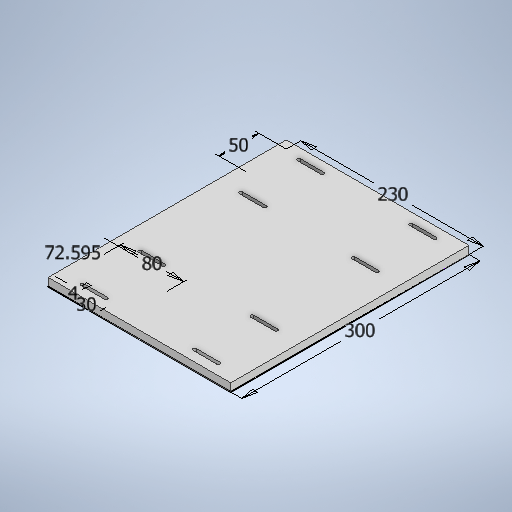
# Autodesk Inventor part: base
Saved by Autodesk Inventor 2025.3 (Build 293356030, 356C)
## iProperties
Created: 2026-06-25
Part Number: base
Material: Generic
Document SubType Name: Modeling
Designer: user
Density: 1 g/cm^3
Appearance: Default
Author: user
Autodesk Inventor part; units mm, degrees
ref_plane "YZ Plane" through (0, 0, 0) normal (1, 0, 0) x (0, 1, 0)
ref_plane "XZ Plane" through (0, 0, 0) normal (0, 1, 0) x (-1, 0, 0)
ref_plane "XY Plane" through (0, 0, 0) normal (0, 0, 1) x (1, 0, 0)
sketch "Sketch1" plane through (0, 0, 0) normal (0, 1, 0) x (-1, 0, 0)
  line L0 (0, 0) -> (-230, 0)
  line L1 (-230, 0) -> (-230, -300)
  line L2 (-230, -300) -> (0, -300)
  line L3 (0, -300) -> (0, 0)
  line L4 (-115, 0) -> (-115, -300) construction
  line L5 (-230, -150) -> (0, -150) construction
  line L6 (0, -250) -> (-230, -250) construction
  line L7 (0, -28.043) -> (0, -96.333) construction
  line L8 (0, -69) -> (0, -31) construction
  line L9 (0, -50) -> (-230, -50) construction
  line L10 (0, -31) -> (-80, -31) construction
  line L11 (-80, -31) -> (-80, -69) construction
  line L12 (-80, -69) -> (0, -69) construction
  line L13 (0, -69) -> (0, -31)
  line L14 (-40, -50) -> (-40, -10.0475) construction
  line L15 (-40, -13.7025) -> (-29.2216, -13.7025)
  line L16 (-40, -13.7025) -> (-59.2216, -13.7025)
  line L17 (-29.2216, -13.7025) -> (-59.2216, -13.7025) construction
  line L18 (-29.2216, -11.7025) -> (-59.2216, -11.7025)
  line L19 (-59.2216, -15.7025) -> (-29.2216, -15.7025)
  arc A0 (-29.2216, -15.7025) -> (-29.2216, -11.7025) centre (-29.2216, -13.7025) ccw
  arc A1 (-59.2216, -11.7025) -> (-59.2216, -15.7025) centre (-59.2216, -13.7025) ccw
  line L20 (-40, -86.2975) -> (-29.2216, -86.2975)
  line L21 (-40, -86.2975) -> (-59.2216, -86.2975)
  line L22 (-29.2216, -86.2975) -> (-59.2216, -86.2975) construction
  line L23 (-29.2216, -88.2975) -> (-59.2216, -88.2975)
  line L24 (-59.2216, -84.2975) -> (-29.2216, -84.2975)
  arc A2 (-29.2216, -88.2975) -> (-29.2216, -84.2975) centre (-29.2216, -86.2975) ccw
  arc A3 (-59.2216, -84.2975) -> (-59.2216, -88.2975) centre (-59.2216, -86.2975) ccw
  line L25 (-230, -31) -> (-150, -31) construction
  line L26 (-150, -31) -> (-150, -69) construction
  line L27 (-150, -69) -> (-230, -69) construction
  line L28 (-190, -13.7025) -> (-200.7784, -13.7025)
  line L29 (-190, -13.7025) -> (-170.7784, -13.7025)
  line L30 (-200.7784, -13.7025) -> (-170.7784, -13.7025) construction
  line L31 (-200.7784, -11.7025) -> (-170.7784, -11.7025)
  line L32 (-170.7784, -15.7025) -> (-200.7784, -15.7025)
  arc A4 (-200.7784, -11.7025) -> (-200.7784, -15.7025) centre (-200.7784, -13.7025) ccw
  arc A5 (-170.7784, -15.7025) -> (-170.7784, -11.7025) centre (-170.7784, -13.7025) ccw
  arc A6 (-170.7784, -88.2975) -> (-170.7784, -84.2975) centre (-170.7784, -86.2975) ccw
  line L33 (-190, -86.2975) -> (-170.7784, -86.2975)
  line L34 (-170.7784, -84.2975) -> (-200.7784, -84.2975)
  line L35 (-190, -86.2975) -> (-200.7784, -86.2975)
  line L36 (-200.7784, -86.2975) -> (-170.7784, -86.2975) construction
  line L37 (-200.7784, -88.2975) -> (-170.7784, -88.2975)
  arc A7 (-200.7784, -84.2975) -> (-200.7784, -88.2975) centre (-200.7784, -86.2975) ccw
  line L38 (-115, -300) -> (-115, 0) construction
  line L39 (0, -250) -> (-230, -250) construction
  line L40 (0, -269) -> (-80, -269) construction
  line L41 (-80, -269) -> (-80, -231) construction
  line L42 (-80, -231) -> (0, -231) construction
  line L43 (-40, -250) -> (-40, -289.9525) construction
  line L44 (-40, -286.2975) -> (-29.2216, -286.2975)
  line L45 (-40, -286.2975) -> (-59.2216, -286.2975)
  line L46 (-29.2216, -286.2975) -> (-59.2216, -286.2975) construction
  line L47 (-29.2216, -288.2975) -> (-59.2216, -288.2975)
  line L48 (-59.2216, -284.2975) -> (-29.2216, -284.2975)
  arc A8 (-29.2216, -288.2975) -> (-29.2216, -284.2975) centre (-29.2216, -286.2975) ccw
  arc A9 (-59.2216, -284.2975) -> (-59.2216, -288.2975) centre (-59.2216, -286.2975) ccw
  arc A10 (-59.2216, -211.7025) -> (-59.2216, -215.7025) centre (-59.2216, -213.7025) ccw
  line L49 (-40, -213.7025) -> (-59.2216, -213.7025)
  line L50 (-59.2216, -215.7025) -> (-29.2216, -215.7025)
  line L51 (-40, -213.7025) -> (-29.2216, -213.7025)
  line L52 (-29.2216, -213.7025) -> (-59.2216, -213.7025) construction
  line L53 (-29.2216, -211.7025) -> (-59.2216, -211.7025)
  arc A11 (-29.2216, -215.7025) -> (-29.2216, -211.7025) centre (-29.2216, -213.7025) ccw
  line L54 (-150, -269) -> (-150, -231) construction
  line L55 (-170.7784, -284.2975) -> (-200.7784, -284.2975)
  line L56 (-190, -286.2975) -> (-200.7784, -286.2975)
  line L57 (-190, -286.2975) -> (-170.7784, -286.2975)
  arc A12 (-200.7784, -284.2975) -> (-200.7784, -288.2975) centre (-200.7784, -286.2975) ccw
  line L58 (-200.7784, -288.2975) -> (-170.7784, -288.2975)
  arc A13 (-170.7784, -288.2975) -> (-170.7784, -284.2975) centre (-170.7784, -286.2975) ccw
  line L59 (-200.7784, -286.2975) -> (-170.7784, -286.2975) construction
  line L60 (-170.7784, -215.7025) -> (-200.7784, -215.7025)
  line L61 (-190, -213.7025) -> (-200.7784, -213.7025)
  arc A14 (-200.7784, -211.7025) -> (-200.7784, -215.7025) centre (-200.7784, -213.7025) ccw
  line L62 (-200.7784, -213.7025) -> (-170.7784, -213.7025) construction
  line L63 (-200.7784, -211.7025) -> (-170.7784, -211.7025)
  line L64 (-190, -213.7025) -> (-170.7784, -213.7025)
  arc A15 (-170.7784, -215.7025) -> (-170.7784, -211.7025) centre (-170.7784, -213.7025) ccw
  line L65 (-150, -231) -> (-230, -231) construction
  line L66 (-230, -269) -> (-150, -269) construction
  point P0 (-40, -31)
  point P1 (-44.2216, -13.7025)
  point P2 (-44.2216, -86.2975)
  point P3 (-190, -50)
  point P4 (-190, -31)
  point P5 (-185.7784, -13.7025)
  point P6 (-185.7784, -86.2975)
  point P7 (-40, -269)
  point P8 (-44.2216, -286.2975)
  point P9 (-44.2216, -213.7025)
  point P10 (-190, -250)
  point P11 (-190, -269)
  point P12 (-185.7784, -213.7025)
  point P13 (-185.7784, -286.2975)
  point P14 (-115, -5)
  point P15 (-44.2216, -86.2975)
  dimension "d0" = 230
  dimension "d1" = 300
  dimension "d5" = 50
  dimension "d15" = 80
  dimension "d25" = 4
  dimension "d33" = 72.595
  dimension "d34" = 30
  constraints: 150 end point, 77 symmetric about line, 32 point on circle, 16 centre point, 10 point on line, 8 midpoint, 5 parallel, 4 horizontal, 4 perpendicular, 4 tangent, 1 collinear, 1 vertical, 14 other
  measures "d0" distance of L2.end L1.end
  measures "d1" distance of L1.end L0.end
  measures "d5" distance between parallel lines of L2 L6
  measures "d15" distance of L12.end L11.end
  measures "d25" distance of L19.end L18.start
  measures "d33" distance between parallel lines of L19 L23
  measures "d34" distance of L16.end L15.end
extrude "Extrusion1" add sketch "Sketch1" along normal blind 10 contours L3 L2 L1 L0 | A0 L19 A1 L18 | L23 A3 L24 A2 | L31 A5 L32 A4 | L37 A7 L34 A6 | L47 A9 L48 A8 | L53 A11 L50 A10 | A13 L58 A12 L55 | L60 A14 L63 A15
extrude "Extrusion2" cut sketch "Sketch1" along normal blind 10 contours A0 L19 A1 L18 | L23 A3 L24 A2 | L31 A5 L32 A4 | L37 A7 L34 A6 | L47 A9 L48 A8 | L53 A11 L50 A10 | A13 L58 A12 L55 | L60 A14 L63 A15
body "Solid1"
